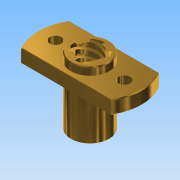
# Autodesk Inventor part: screw t8
Saved by Autodesk Inventor 2017 (Build 210142000, 142)
## iProperties
Part Number: screw t8
Material: Типовые
Document SubType Name: Modeling
Designer: alcapone
Density: 1 g/cm^3
Appearance: Латунь - сатинированная
Mass: 1.43597 g
Surface Area: 19.8056 cm^2
Volume: 1.43597 cm^3
Author: alcapone
Autodesk Inventor part; units mm, degrees
ref_plane "YZ Plane" through (0, 0, 0) normal (1, 0, 0) x (0, 1, 0)
ref_plane "XZ Plane" through (0, 0, 0) normal (0, 1, 0) x (-1, 0, 0)
ref_plane "XY Plane" through (0, 0, 0) normal (0, 0, 1) x (1, 0, 0)
sketch "Эскиз6" plane through (0, 0, 0) normal (0, 0, 1) x (1, 0, 0)
  arc A0 (11.7132, -6.3) -> (11.7132, 6.3) centre (1.5, 0) ccw
  line L0 (11.7132, 6.3) -> (-11.7132, 6.3)
  arc A1 (-11.7132, 6.3) -> (-11.7132, -6.3) centre (-1.5, 0) ccw
  line L1 (-11.7132, -6.3) -> (11.7132, -6.3)
  circle A2 centre (-9, 0) radius 1.5
  circle A3 centre (9, 0) radius 1.5
  circle A4 centre (0, 0) radius 5
  circle A5 centre (0, 0) radius 5
  circle A6 centre (0, 0) radius 4
  circle A7 centre (0, 0) radius 3
  dimension "d23" = 6
  constraints: 8 centre point, 4 end point, 4 point on circle, 1 coincident
  measures "d23" diameter of A7
extrude "Выдавливание4" add sketch "Эскиз6" along normal blind 3.5 contours L1 A1 L0 A0 | A4
extrude "Выдавливание5" add sketch "Эскиз6" against normal blind 12 contours A4 | A6
extrude "Выдавливание6" add sketch "Эскиз6" along normal blind 5.5 contours A4 | A6
sketch "Эскиз2" plane through (0, 0, 0) normal (0, 0, 1) x (1, 0, 0)
  circle A0 centre (0, 0) radius 4
  dimension "d0" = 8
  constraints: 1 centre point, 1 coincident
  measures "d0" diameter of A0
sketch "Эскиз7" plane through (0, 0, 0) normal (0, 1, 0) x (-1, 0, 0)
  line L0 (0, -13.5272) -> (0, 21.8679) construction
  line L1 (0, -13.5272) -> (5.4466, -13.5272) construction
  line L2 (4, -13.5272) -> (3, -13.5272)
  line L3 (3, -13.5272) -> (3, -12.5272)
  line L4 (3, -12.5272) -> (4, -12.5272)
  line L5 (4, -12.5272) -> (4, -13.5272)
  point P0 (0, 0)
  dimension "d30" = 1
  dimension "d31" = 1
  dimension "d32" = 3
  constraints: 12 end point, 2 horizontal, 2 parallel, 1 perpendicular, 1 point on line, 1 vertical
  measures "d30" distance between parallel lines of L1 L4
  measures "d31" distance between parallel lines of L3 L5
  measures "d32" distance between parallel lines of L0 L3
coil "Пружина2" sketch "Эскиз7" operation cut axis through (0, 0, -13.5272) along (0, 0, 1) pitch 8 turns 4 hand right
pattern_circular "Круговой массив2" count 4 over 360 about axis through (0, 0, 0) along (0, 0, -1) of "Пружина2"
chamfer "Фаска1" distance 0.2 angle 45 2 edges at (-5, 0, 5.5) (-5, 0, -12)
chamfer "Фаска2" distance 0.2 angle 45 8 edges at (-13.5, 0, 3.5) (0, 6.3, 3.5) (0, -6.3, 3.5) (13.5, 0, 3.5) (0, -6.3, 0) (13.5, 0, 0) (0, 6.3, 0) (-13.5, 0, 0)
sketch "Эскиз8" plane through (-11.7132, 6.3, 0.2) normal (0, 1, 0) x (1, 0, 0)
  line L0 (11.7132, 0.2) -> (11.7132, 23.6833)
  line L1 (9.7132, 15.8196) -> (13.7132, 15.8196)
  line L2 (13.7132, 15.8196) -> (13.7132, 7.2)
  line L3 (13.7132, 7.2) -> (9.7132, 7.2)
  line L4 (9.7132, 7.2) -> (9.7132, 15.8196)
  line L5 (6.9132, 12.2) -> (16.5132, 12.2) projected
  dimension "d50" = 4
  dimension "d51" = 5
  constraints: 10 end point, 2 parallel, 1 horizontal, 1 perpendicular, 1 vertical, 1 other
  measures "d50" distance between parallel lines of L2 L4
  measures "d51" distance between parallel lines of L5 L3
extrude "Выдавливание7" cut sketch "Эскиз8" against normal blind 30
